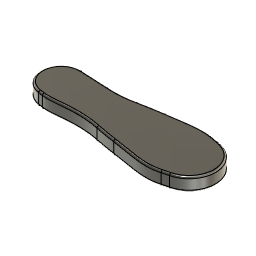
3-braco v1 (Autodesk Fusion 360 design; units mm, degrees)
Autodesk Fusion 360 part; units mm, degrees
sketch "Sketch2" plane through (0, 0, 0) normal (0, 0, 1) x (1, 0, 0)
  line L0 (50, 150) -> (50, -70) construction
  line L1 (250, 90.0697) -> (250, 10.6987) construction
  arc A0 (52.3019, 80.7374) -> (46.7232, 21.0708) centre (50.9864, 50.7663) ccw
  arc A1 (254.3659, 11.4976) -> (254.1757, 89.3161) centre (244.994, 50.3842) ccw
  line L2 (250, 10.6987) -> (0, 10.6987) construction
  line L3 (250, 90.0697) -> (0, 90.0697) construction
  line L4 (150, 150) -> (150, -50) construction
  line L5 (150, 85.4099) -> (0, 85.4099) construction
  line L6 (150, 15.7406) -> (0, 15.7406) construction
  spline S0 degree 3 poles (94.5111, 78.6458) (106.2581, 77.9971) (119.8362, 78.3242) (135.6331, 81.6704) knots 0.557908 0.557908 0.557908 0.557908 0.900334 0.900334 0.900334 0.900334
  spline S1 degree 3 poles (171.2576, 87.8799) (203.5545, 92.3128) (221.7309, 97.5645) (248.6541, 90.6737) knots 0.155993 0.155993 0.155993 0.155993 0.934704 0.934704 0.934704 0.934704
  spline S2 degree 3 poles (53.4006, 20.106) (71.1646, 17.523) (97.3135, 27.0878) (137.1784, 18.8893) knots 0.056296 0.056296 0.056296 0.056296 0.911507 0.911507 0.911507 0.911507
  spline S3 degree 3 poles (167.9292, 13.5597) (202.4371, 8.6827) (220.9926, 2.4041) (244.2709, 8.8782) knots 0.129297 0.129297 0.129297 0.129297 0.935081 0.935081 0.935081 0.935081
  arc A2 (137.1784, 18.8893) -> (167.9292, 13.5597) centre (237.8982, 508.6398) ccw
  arc A3 (171.2576, 87.8799) -> (135.6331, 81.6704) centre (239.2472, -407.4759) ccw
  arc A4 (248.6541, 90.6737) -> (254.1757, 89.3161) centre (323.0387, 381.3057) ccw
  line L7 (171.2576, 87.8799) -> (203.5545, 92.3128)
  line L8 (203.5545, 92.3128) -> (221.7309, 97.5645)
  line L9 (221.7309, 97.5645) -> (248.6541, 90.6737)
  arc A5 (254.3659, 11.4976) -> (244.2709, 8.8782) centre (324.6549, -280.1519) ccw
  line L10 (167.9292, 13.5597) -> (202.4371, 8.6827)
  line L11 (202.4371, 8.6827) -> (220.9926, 2.4041)
  line L12 (220.9926, 2.4041) -> (244.2709, 8.8782)
  arc A6 (53.4006, 20.106) -> (46.7232, 21.0708) centre (-484.7592, -3680.9728) ccw
  line L13 (53.4006, 20.106) -> (71.1646, 17.523)
  line L14 (71.1646, 17.523) -> (97.3135, 27.0878)
  line L15 (97.3135, 27.0878) -> (137.1784, 18.8893)
  arc A7 (94.5111, 78.6458) -> (52.3019, 80.7374) centre (-111.699, -3655.6651) ccw
  line L16 (94.5111, 78.6458) -> (106.2581, 77.9971)
  line L17 (106.2581, 77.9971) -> (119.8362, 78.3242)
  line L18 (119.8362, 78.3242) -> (135.6331, 81.6704)
  dimension "d8" = 200
  dimension "d9" = 30
  dimension "d10" = 40
  dimension "d15" = 500
  dimension "d16" = 500
  dimension "d17" = 300
  dimension "d18" = 300
  dimension "d21" = 3740
  dimension "d22" = 3740
  constraint perpendicular L0 L2
  constraint perpendicular L0 L3
  constraint vertical L4
  constraint perpendicular L0 L5
  constraint perpendicular L0 L6
  constraint tangent S3 A2
  constraint tangent S2 A2
  constraint tangent S0 A3
  constraint tangent S1 A3
  constraint tangent S1 A4
  constraint tangent A1 A4
  constraint tangent S3 A5
  constraint tangent A1 A5
  constraint tangent A0 A6
  constraint tangent S2 A6
  constraint tangent A0 A7
  constraint tangent S0 A7
  measures "d8" distance of L0 L1
  measures "d9" radius of A0
  measures "d10" radius of A1
  measures "d15" radius of A2
  measures "d16" radius of A3
  measures "d17" radius of A4
  measures "d18" radius of A5
  measures "d21" radius of A6
  measures "d22" radius of A7
extrude "Extrude1" add sketch "Sketch2" along normal blind 20 contours A0 A1 S1 S2 S3 A2 A3 A4 L7 L8 A5 L10 L11 A6 L14 L15 A7 L16 L17 L18 | S0 L16 L17 L18 | S2 L14 L15 | S1 L7 L8 | S3 L10 L11
fillet "Fillet1" radius 2.5 6 edges at (21.1167, 53.5591, 20) (87.0017, 21.6034, 20) (210.3111, 6.9623, 20) (284.9939, 50.4819, 20) (211.971, 93.5232, 20) (113.5534, 78.66, 20)
fillet "Fillet2" radius 2.5 10 edges at (21.1167, 53.5591, 0) (87.0017, 21.6034, 0) (152.5122, 15.9845, 0) (210.3111, 6.9623, 0) (249.307, 10.2318, 0) (284.9939, 50.4819, 0) (251.4117, 89.9818, 0) (211.971, 93.5232, 0) (153.3892, 85.0974, 0) (113.5534, 78.66, 0)
